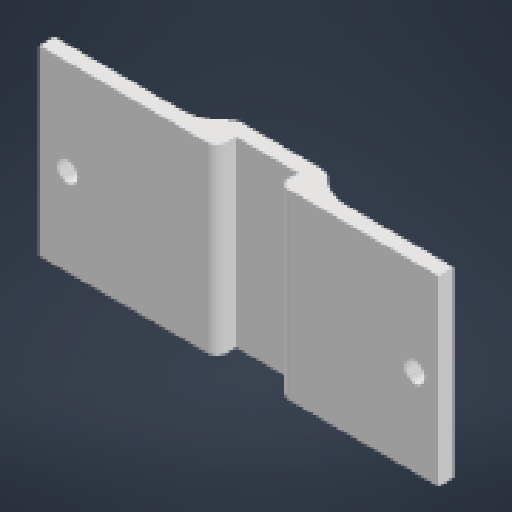
# Autodesk Inventor part: драйвер 2
Saved by Autodesk Inventor 2025 (Build 290162000, 162)
## iProperties
Created: 2025-03-13
Part Number: драйвер 2
Material: Типовые
Document SubType Name: Modeling
Designer: Phantom
Density: 1 g/cm^3
Appearance: По умолчанию
Author: Phantom
Autodesk Inventor part; units mm, degrees
note: some values were not read from the file. Chosen so that the rebuilt part matches the saved one: edges of "Сопряжение1".
ref_plane "YZ Plane" through (0, 0, 0) normal (1, 0, 0) x (0, 1, 0)
ref_plane "XZ Plane" through (0, 0, 0) normal (0, 1, 0) x (-1, 0, 0)
ref_plane "XY Plane" through (0, 0, 0) normal (0, 0, 1) x (1, 0, 0)
sketch "Эскиз1" plane through (0, 0, 0) normal (0, 0, 1) x (1, 0, 0)
  line L0 (-52.8161, -17.6697) -> (52.3618, -17.6697)
  line L1 (-52.8161, 20.3303) -> (52.3618, 20.3303)
  line L2 (52.3618, 20.3303) -> (52.3618, -17.6697)
  line L3 (52.3618, -17.6697) -> (-52.8161, -17.6697)
  line L4 (-52.8161, -17.6697) -> (-52.8161, 20.3303)
  circle A0 centre (-47.8161, 0.5303) radius 2.1
  circle A1 centre (47.3618, 0.5303) radius 2.1
  point P0 (0, 0)
  point P1 (-8.6177, 20.3303)
  constraints: 10 end point, 2 centre point, 2 parallel, 1 horizontal, 1 perpendicular
extrude "Выдавливание1" add sketch "Эскиз1" along normal blind 3.2
sketch "Эскиз2" plane through (-52.8161, -17.6697, 0) normal (0, -1, 0) x (1, 0, 0)
  line L0 (105.1779, 3.2) -> (0, 3.2) projected
  line L1 (105.1779, 0) -> (0, 0) projected
  line L2 (72, 3.2) -> (59, 3.2)
  line L3 (59, 3.2) -> (59, 0)
  line L4 (59, 0) -> (72, 0)
  line L5 (72, 3.2) -> (59, 3.2)
  line L6 (59, 3.2) -> (59, -0.8)
  line L7 (59, -0.8) -> (72, -0.8)
  line L8 (72, -0.8) -> (72, 3.2)
  point P0 (52.8161, 0)
  dimension "d5" = 4
  constraints: 14 end point, 3 parallel, 3 point on line, 2 horizontal, 2 perpendicular
  measures "d5" distance of L7.end L2.start
extrude "Выдавливание2" cut sketch "Эскиз2" against normal through all
fillet "Сопряжение1" radius 2 1 edges at (6.1839, 1.3303, 3.2)
sketch "Эскиз3" plane through (-52.8161, -17.6697, 0) normal (0, -1, 0) x (1, 0, 0)
  line L0 (105.1779, 3.2) -> (72, 3.2) projected
  line L1 (72, 3.2) -> (59, 3.2)
  line L2 (59, 3.2) -> (59, -0.8)
  line L3 (59, -0.8) -> (72, -0.8)
  line L4 (72, -0.8) -> (72, 3.2)
  line L5 (72, -0.8) -> (59, -0.8)
  line L6 (59, -0.8) -> (59, -4)
  line L7 (59, -4) -> (72, -4)
  line L8 (72, -4) -> (72, -0.8)
  line L9 (72, 0) -> (105.1779, 0) projected
  line L10 (72, -4) -> (75.2, -4)
  line L11 (75.2, -4) -> (75.2, 0)
  line L12 (75.2, 0) -> (72, 0)
  line L13 (72, 0) -> (72, -4)
  line L14 (59, -4) -> (55.8, -4)
  line L15 (55.8, -4) -> (55.8, 0)
  line L16 (55.8, 0) -> (59, 0)
  line L17 (59, 0) -> (59, -4)
  point P0 (52.8161, 0)
  dimension "d6" = 13
  dimension "d7" = 4
  dimension "d8" = 13
  dimension "d9" = 3.2
  dimension "d10" = 3.2
  dimension "d11" = 3.2
  constraints: 32 end point, 8 parallel, 4 horizontal, 4 perpendicular, 2 point on line
  measures "d6" distance of L3.end L2.end
  measures "d7" distance of L2.end L1.end
  measures "d8" distance of L7.end L6.end
  measures "d9" distance of L6.end L5.end
  measures "d10" distance of L12.end L11.end
  measures "d11" distance of L15.end L16.end
extrude "Выдавливание3" add sketch "Эскиз3" against normal up to surface (38 mm away) contours L9 L11 L10 L8 L4 | L2 L6 L14 L15 L16 | L8 L7 L6 L3
fillet "Сопряжение2" radius 2 1 edges at (19.1839, 1.3303, 3.2)
fillet "Сопряжение3" radius 9 2 edges at (22.3839, 1.3303, 0) (2.9839, 1.3303, 0)
fillet "Сопряжение4" radius 3.25 2 edges at (2.9839, 1.3303, -4) (22.3839, 1.3303, -4)
sketch "Эскиз4" plane through (0, 0, 0) normal (0, 0, -1) x (-1, 0, 0)
  line L0 (30.891, 20.3303) -> (19.391, 20.3303) projected
  line L1 (30.891, -17.6697) -> (30.891, 20.3303) projected
  line L2 (19.391, -17.6697) -> (30.891, -17.6697) projected
  line L3 (19.391, -17.6697) -> (19.391, 20.3303) projected
  circle A0 centre (24.991, 0.5303) radius 2.1 projected
  line L4 (4.4994, -17.6697) -> (4.4994, 20.3303) projected
  line L5 (52.8161, -17.6697) -> (4.4994, -17.6697) projected
  line L6 (52.8161, 20.3303) -> (52.8161, -17.6697) projected
  line L7 (4.4994, 20.3303) -> (52.8161, 20.3303) projected
  circle A1 centre (47.8161, 0.5303) radius 2.1 projected
  point P0 (0, 0)
extrude "Выдавливание4" cut sketch "Эскиз4" against normal blind 10 contours L7 L6 L5 L1 | A0
